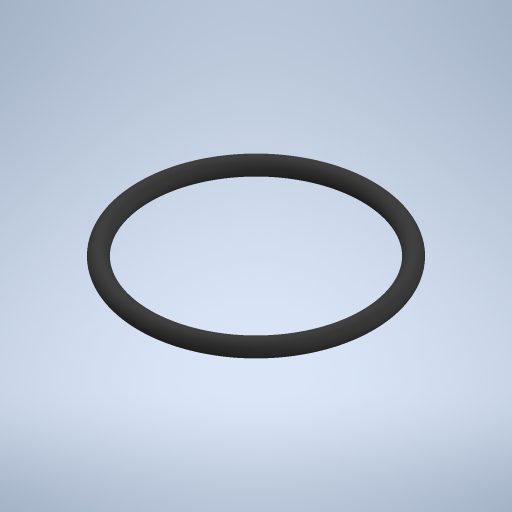
# Autodesk Inventor part: ORing 222 G40
Saved by Autodesk Inventor 2023.2 (Build 272271000, 271)
## iProperties
Created: 2023-06-22
Part Number: ORing 222 G40
Material: Rubber
Document SubType Name: Modeling
Designer: Nathan Cai
Density: 0.93 g/cm^3
Appearance: Rubber - Black
Author: Nathan Cai
Autodesk Inventor part; units mm, degrees
ref_plane "YZ Plane" through (0, 0, 0) normal (1, 0, 0) x (0, 1, 0)
ref_plane "XZ Plane" through (0, 0, 0) normal (0, 1, 0) x (-1, 0, 0)
ref_plane "XY Plane" through (0, 0, 0) normal (0, 0, 1) x (1, 0, 0)
sketch "Sketch1" plane through (0, 0, 0) normal (0, 0, 1) x (1, 0, 0)
  line L0 (0, 0) -> (19.7, 0) construction
  circle A0 centre (21.25, 0) radius 1.55
  line L1 (0, 0) -> (0, 6.35) construction
  point P0 (22.8, 0)
  dimension "d0" = 19.7
  dimension "d1" = 3.1
  dimension "d2" = 6.35
  constraints: 4 end point, 2 point on circle, 1 centre point, 1 horizontal, 1 point on line, 1 vertical
  measures "d0" distance of L0.start L0.end
  measures "d1" diameter of A0
  measures "d2" distance of L0.start L1.end
revolve "Revolution1" add sketch "Sketch1" angle 360 about axis through (0, 0, 0) along (0, 1, 0)
body "Solid1"
